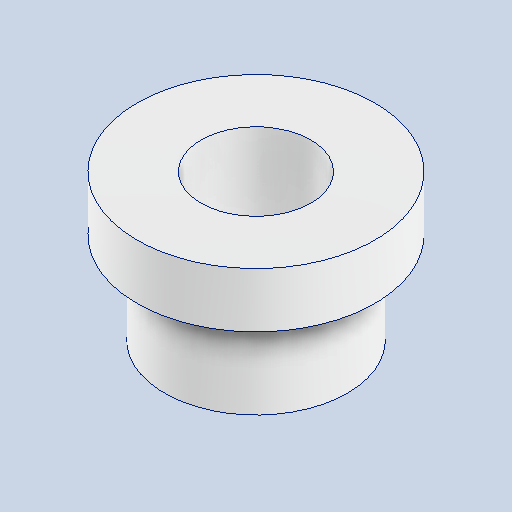
# Autodesk Inventor part: 1173
Saved by Autodesk Inventor 2025.1 (Build 291241000, 241)
## iProperties
Created: 2024-06-11
Part Number: 1173
Material: Aluminium 6061
Document SubType Name: Modeling
Designer: ffogue
Density: 2.7 g/cm^3
Appearance: Aluminium - flach
Author: ffogue
Autodesk Inventor part; units mm, degrees
ref_plane "YZ Plane" through (0, 0, 0) normal (1, 0, 0) x (0, 1, 0)
ref_plane "XZ Plane" through (0, 0, 0) normal (0, 1, 0) x (-1, 0, 0)
ref_plane "XY Plane" through (0, 0, 0) normal (0, 0, 1) x (1, 0, 0)
sketch "Skizze1" plane through (0, 0, 0) normal (0, 1, 0) x (-1, 0, 0)
  line L0 (0, 0) -> (6.5, 0)
  line L1 (6.5, 0) -> (6.5, -3)
  line L2 (6.5, -3) -> (5, -3)
  line L3 (5, -3) -> (5, -8)
  line L4 (5, -8) -> (0, -8)
  line L5 (0, -8) -> (0, 0)
  point P0 (5.75, -3)
  dimension "d0" = 3
  dimension "d1" = 5
  dimension "d2" = 10
  dimension "d3" = 13
  constraints: 12 end point, 5 perpendicular, 1 horizontal, 1 midpoint
  measures "d0" distance between parallel lines of L2 L0
  measures "d1" distance from line of L4 point (5.75, -3)
  measures "d2" diameter of L3 L5
  measures "d3" diameter of L1 L5
revolve "Umdrehung1" add sketch "Skizze1" angle 360 about axis through (0, 0, -8) along (0, 0, 1)
sketch "Skizze2" plane through (0, 0, 0) normal (0, 0, 1) x (1, 0, 0)
  circle A0 centre (0, 0) radius 6.5 projected
  point P0 (0, 0)
  constraints: 1 coincident
hole "Bohrung1" at (0, 0, 0) direction (0, 0, -1) diameter 6 end through all
